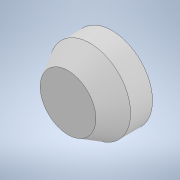
# Autodesk Inventor part: GehaeuseteilB
Saved by Autodesk Inventor 2020.2 (Build 242310000, 310)
## iProperties
Created: 2020-02-12
Part Number: GehaeuseteilB
Material: Generisch
Document SubType Name: Modeling
Designer: Max
Density: 1 g/cm^3
Appearance: Vorgabe
Author: Max
Autodesk Inventor part; units mm, degrees
ref_plane "YZ Plane" through (0, 0, 0) normal (1, 0, 0) x (0, 1, 0)
ref_plane "XZ Plane" through (0, 0, 0) normal (0, 1, 0) x (-1, 0, 0)
ref_plane "XY Plane" through (0, 0, 0) normal (0, 0, 1) x (1, 0, 0)
sketch "Skizze2" plane through (0, 0, 0) normal (0, 1, 0) x (-1, 0, 0)
  line L0 (-60, -3) -> (60, -3) projected
  line L1 (60, 0) -> (60, -3)
  line L2 (-60, 0) -> (60, 0) projected
  line L3 (-60, 0) -> (-60, -3)
  line L4 (1.7274, 123.0345) -> (1.7274, -32.1262)
  line L5 (60, 0) -> (60, 31.4988)
  line L6 (60, 31.4988) -> (41.7274, 63.1479)
  line L7 (41.7274, 63.1479) -> (1.7274, 63.1479)
  line L8 (1.7274, 63.1479) -> (1.7274, 58.1479)
  line L9 (39.6141, 58.1479) -> (1.7274, 58.1479)
  line L10 (39.6141, 58.1479) -> (55, 31.4988)
  line L11 (55, 31.4988) -> (55, 0)
  line L12 (60, 0) -> (55, 0)
  point P0 (0, 0)
  dimension "d0" = 31.4988
  dimension "d1" = 150
  dimension "d2" = 40
  dimension "d4" = 31.6491
  dimension "d5" = 150
  dimension "d6" = 5
  dimension "d7" = 5
  constraints: 22 end point, 4 vertical, 3 perpendicular, 3 point on line, 2 parallel, 1 collinear, 1 other
  measures "d0" distance of L1.start L5.end
  measures "d1" angle of L5 L6
  measures "d2" distance of L6.end L7.end
  measures "d4" vertical distance of L5.end L6.end
  measures "d5" angle of L10 L11
  measures "d6" distance between parallel lines of L11 L5
  measures "d7" distance between parallel lines of L7 L9
revolve "Umdrehung1" add sketch "Skizze2" angle 360 about axis through (-1.7274, 0, 123.0345) along (0, 0, -1) contours L2 L11 L10 L9 L4 L7 L6 L5
